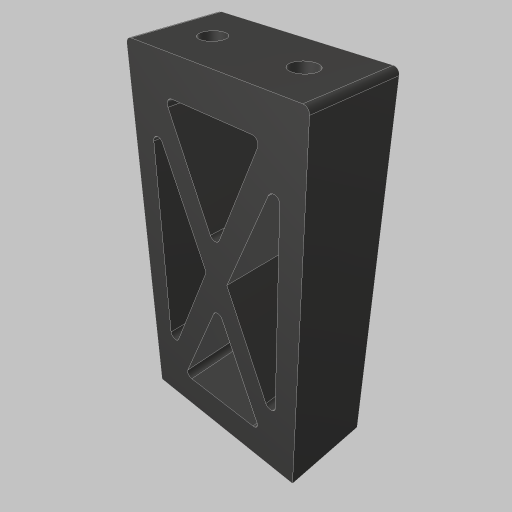
# Autodesk Inventor part: DB1-024
Saved by Autodesk Inventor 2023.5 (Build 275446000, 446)
## iProperties
Created: 2025-03-10
Part Number: DB1-024
Material: ABS Plastic
Document SubType Name: Modeling
Designer: brand
Density: 1.06 g/cm^3
Appearance: Smooth - Black
Author: brand
Autodesk Inventor part; units mm, degrees
ref_plane "YZ Plane" through (0, 0, 0) normal (1, 0, 0) x (0, 1, 0)
ref_plane "XZ Plane" through (0, 0, 0) normal (0, 1, 0) x (-1, 0, 0)
ref_plane "XY Plane" through (0, 0, 0) normal (0, 0, 1) x (1, 0, 0)
sketch "Sketch1" plane through (0, 0, 0) normal (0, 1, 0) x (-1, 0, 0)
  line L0 (25.4, 12.7) -> (-25.4, 12.7)
  line L1 (-25.4, 12.7) -> (-25.4, -12.7)
  line L2 (-25.4, -12.7) -> (25.4, -12.7)
  line L3 (25.4, -12.7) -> (25.4, 12.7)
  line L4 (25.4, 12.7) -> (-25.4, -12.7) construction
  line L5 (-25.4, 12.7) -> (25.4, -12.7) construction
  point P0 (0, 0)
  dimension "d0" = 50.8
  dimension "d1" = 25.4
  constraints: 12 end point, 2 midpoint, 2 parallel, 1 horizontal, 1 perpendicular
  measures "d0" distance of L2.end L1.end
  measures "d1" distance of L1.end L0.end
extrude "Extrusion1" add sketch "Sketch1" along normal mid plane 99.06
sketch "Sketch2" plane through (-25.4, 49.53, 12.7) normal (0, 0, 1) x (1, 0, 0)
  line L0 (50.8, -99.06) -> (0, -99.06) construction
  line L1 (0, -99.06) -> (0, 0) construction
  line L2 (0, 0) -> (50.8, 0) construction
  line L3 (50.8, 0) -> (50.8, -99.06) construction
  line L4 (44.45, -6.35) -> (6.35, -6.35) construction
  line L5 (6.35, -6.35) -> (6.35, -92.71) construction
  line L6 (6.35, -92.71) -> (44.45, -92.71) construction
  line L7 (44.45, -92.71) -> (44.45, -6.35) construction
  line L8 (6.35, -6.35) -> (44.45, -92.71) construction
  line L9 (6.35, -92.71) -> (44.45, -6.35) construction
  line L10 (6.35, -14.2159) -> (40.9797, -92.71) construction
  line L11 (44.45, -84.8441) -> (9.8203, -6.35) construction
  line L12 (40.9797, -6.35) -> (6.35, -84.8441) construction
  line L13 (9.8203, -92.71) -> (44.45, -14.2159) construction
  line L14 (0, -99.06) -> (0, 0) construction
  line L15 (0, -89.281) -> (50.8, -89.281) construction
  line L16 (50.8, -99.06) -> (50.8, 0) construction
  line L17 (25.4, -57.3959) -> (11.3331, -89.281)
  line L18 (11.3331, -89.281) -> (39.4669, -89.281)
  line L19 (39.4669, -89.281) -> (25.4, -57.3959)
  line L20 (28.8703, -49.53) -> (44.45, -84.8441)
  line L21 (44.45, -84.8441) -> (44.45, -14.2159)
  line L22 (44.45, -14.2159) -> (28.8703, -49.53)
  line L23 (9.8203, -6.35) -> (25.4, -41.6641)
  line L24 (9.8092, -6.35) -> (40.9797, -6.35) construction
  line L25 (40.9797, -6.35) -> (25.4, -41.6641)
  line L26 (6.35, -14.2159) -> (6.35, -84.8441)
  line L27 (6.35, -84.8441) -> (21.9297, -49.53)
  line L28 (21.9297, -49.53) -> (6.35, -14.2159)
  line L29 (0, -9.779) -> (50.8, -9.779) construction
  line L30 (11.3331, -9.779) -> (39.4669, -9.779)
  point P0 (25.4, -49.53)
  point P1 (9.8203, -6.35)
  dimension "d4" = 6.35
  dimension "d5" = 3.175
  dimension "d6" = 3.175
  dimension "d7" = 3.175
  dimension "d8" = 3.175
  dimension "d9" = 9.779
  dimension "d23" = 9.779
  constraints: 50 end point, 29 point on line, 6 collinear, 5 parallel, 3 perpendicular, 3 other
  measures "d4" distance between parallel lines of L2 L4
  measures "d5" distance between parallel lines of L11 L8
  measures "d6" distance between parallel lines of L10 L8
  measures "d7" distance between parallel lines of L9 L12
  measures "d8" distance between parallel lines of L9 L13
  measures "d9" distance between parallel lines of L0 L15
  measures "d23" distance between parallel lines of L2 L29
extrude "Extrusion2" cut sketch "Sketch2" against normal through all
fillet "Fillet1" radius 1.5875 13 edges at (-14.0669, -39.751, 0) (-19.05, -35.3141, 0) (14.0669, -39.751, 0) (19.05, -35.3141, 0) (0, 7.8659, 0) (-3.4703, 0, 0) (-19.05, 35.3141, 0) (19.05, 35.3141, 0) (0, -7.8659, 0) (25.4, 49.53, 0) (-25.4, 49.53, 0) (-14.0669, 39.751, 0) (14.0669, 39.751, 0)
sketch "Sketch3" plane through (0, -49.53, 0) normal (0, -1, 0) x (1, 0, 0)
  line L0 (-25.4, 12.7) -> (25.4, 12.7) construction
  line L1 (25.4, 12.7) -> (25.4, -12.7) construction
  line L2 (25.4, -12.7) -> (-25.4, -12.7) construction
  line L3 (-25.4, -12.7) -> (-25.4, 12.7) construction
  line L4 (-6.35, 0) -> (6.35, 0) construction
  point P0 (0, 0)
  point P1 (0, 0)
  point P2 (-19.05, 0)
  point P3 (19.05, 0)
  dimension "d12" = 12.7
  dimension "d13" = 12.7
  dimension "d14" = 12.7
  constraints: 2 end point, 2 horizontal alignment, 1 coincident, 1 horizontal, 1 midpoint
  measures "d12" distance of L4.end L4.start
  measures "d13" distance of point (-19.05, 0) L4.start
  measures "d14" distance of point (19.05, 0) L4.end
hole "Hole1" at (-6.35, -49.53, 0) at (6.35, -49.53, 0) at (-19.05, -49.53, 0) at (19.05, -49.53, 0) direction (0, 1, 0) diameter 6.75 depth 9.525
sketch "Sketch4" plane through (0, 49.53, 0) normal (0, 1, 0) x (1, 0, 0)
  line L0 (-12.7, 0) -> (12.7, 0) construction
  point P0 (0, 0)
  point P1 (0, 0)
  dimension "d24" = 25.4
  constraints: 3 coincident, 2 end point, 1 horizontal, 1 midpoint
  measures "d24" distance of L0.start L0.end
hole "Hole2" at (-12.7, 49.53, 0) at (12.7, 49.53, 0) direction (0, -1, 0) diameter 6.75 depth 9.525
equation "\"d6\" = d5"
equation "\"d7\" = d5"
equation "\"d8\" = d7"
equation "\"d23\" = d9"
equation "\"d13\" = d12"
equation "\"d14\" = d13"
body "Solid1"
